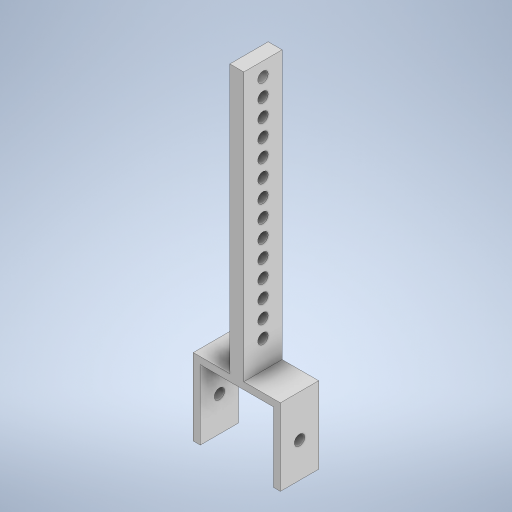
# Autodesk Inventor part: catcher
Saved by Autodesk Inventor 2024 (Build 280153000, 153)
## iProperties
Created: 2024-07-10
Part Number: catcher
Material: 일반
Document SubType Name: Modeling
Designer: Gihyeok Na
Density: 1 g/cm^3
Appearance: 기본값
Author: Gihyeok Na
Autodesk Inventor part; units mm, degrees
ref_plane "YZ Plane" through (0, 0, 0) normal (1, 0, 0) x (0, 1, 0)
ref_plane "XZ Plane" through (0, 0, 0) normal (0, 1, 0) x (-1, 0, 0)
ref_plane "XY Plane" through (0, 0, 0) normal (0, 0, 1) x (1, 0, 0)
sketch "스케치4" plane through (0, 0, 0) normal (0, 1, 0) x (-1, 0, 0)
  line L0 (-2, 5.5) -> (-2, -5.5)
  line L1 (-2, -5.5) -> (2, -5.5)
  line L2 (2, -5.5) -> (2, 5.5)
  line L3 (2, 5.5) -> (-2, 5.5)
  line L4 (-2, 5.5) -> (2, -5.5) construction
  line L5 (-2, -5.5) -> (2, 5.5) construction
  point P0 (0, 0)
  point P1 (0, 0)
  dimension "d12" = 11
  dimension "d13" = 4
  constraints: 12 end point, 3 midpoint, 2 parallel, 1 perpendicular, 1 vertical
  measures "d12" distance of L0.start L0.end
  measures "d13" distance of L1.end L0.end
extrude "돌출3" add sketch "스케치4" along normal blind 77
sketch "스케치5" plane through (0, 0, 0) normal (0, -1, 0) x (1, 0, 0)
  line L0 (-10.5, -5.5) -> (10.5, -5.5)
  line L1 (10.5, -5.5) -> (10.5, 5.5)
  line L2 (10.5, 5.5) -> (-10.5, 5.5)
  line L3 (-10.5, 5.5) -> (-10.5, -5.5)
  line L4 (-10.5, -5.5) -> (10.5, 5.5) construction
  line L5 (10.5, -5.5) -> (-10.5, 5.5) construction
  line L6 (0, 5.5) -> (0, -5.5) construction
  line L7 (10.5, 5.5) -> (12.5, 5.5)
  line L8 (12.5, 5.5) -> (12.5, -5.5)
  line L9 (12.5, -5.5) -> (10.5, -5.5)
  line L10 (-10.5, 5.5) -> (-12.5, 5.5)
  line L11 (-12.5, 5.5) -> (-12.5, -5.5)
  line L12 (-12.5, -5.5) -> (-10.5, -5.5)
  line L13 (-22.4262, 19.8) -> (40.7349, 19.8) construction
  point P0 (0, 0)
  point P1 (0, 0)
  dimension "d16" = 21
  dimension "d17" = 11
  dimension "d18" = 2
  dimension "d43" = 19.8
  constraints: 28 end point, 5 midpoint, 3 horizontal, 3 perpendicular, 2 parallel, 2 symmetric about line
  measures "d16" distance of L0.start L0.end
  measures "d17" distance of L1.end L0.end
  measures "d18" distance of L1.end L7.end
  measures "d43" distance from line of point (0, 0) L13
extrude "돌출4" add sketch "스케치5" along normal blind 2
extrude "돌출5" add sketch "스케치5" along normal blind 22 contours L12 L11 L10 L3 | L1 L7 L8 L9
sketch "스케치6" plane through (-12.5, 0, -5.5) normal (-1, 0, 0) x (0, 0, 1)
  line L0 (11, 0) -> (0, 0) projected
  line L1 (0, 0) -> (0, -22) projected
  line L2 (11, -22) -> (0, -22) projected
  line L3 (11, 0) -> (11, -22) projected
  circle A0 centre (5.5, -12) radius 1.5
  point P0 (5.5, 0)
  dimension "d23" = 3
  dimension "d24" = 10
  constraints: 1 centre point
  measures "d23" diameter of A0
  measures "d24" distance from line of A0.centre L2
extrude "돌출6" cut sketch "스케치6" against normal through all contours A0
sketch "스케치7" plane through (-2, 77, -5.5) normal (-1, 0, 0) x (0, 0, 1)
  line L0 (0, -77) -> (11, -77) projected
  line L1 (11, -77) -> (11, 0) projected
  line L2 (0, 0) -> (11, 0) projected
  line L3 (0, -77) -> (0, 0) projected
  line L4 (0, -73) -> (11, -73) construction
  line L5 (0, -4) -> (11, -4) construction
  line L6 (0, -69) -> (11, -69) construction
  circle A0 centre (5.5, -4) radius 1.5
  circle A1 centre (5.5, -69) radius 1.5
  line L7 (5.5, -69) -> (5.5, -4) construction
  circle A2 centre (5.5, -64) radius 1.5
  circle A3 centre (5.5, -59) radius 1.5
  circle A4 centre (5.5, -54) radius 1.5
  circle A5 centre (5.5, -49) radius 1.5
  circle A6 centre (5.5, -44) radius 1.5
  circle A7 centre (5.5, -39) radius 1.5
  circle A8 centre (5.5, -34) radius 1.5
  circle A9 centre (5.5, -29) radius 1.5
  circle A10 centre (5.5, -24) radius 1.5
  circle A11 centre (5.5, -19) radius 1.5
  circle A12 centre (5.5, -14) radius 1.5
  circle A13 centre (5.5, -9) radius 1.5
  point P0 (5.5, -77)
  dimension "d27" = 4
  dimension "d28" = 4
  dimension "d29" = 4
  dimension "d30" = 3
  dimension "d31" = 5.5
  dimension "d32" = 3
  dimension "d35" = 5
  constraints: 14 centre point, 8 end point, 5 point on line, 4 perpendicular, 2 midpoint, 1 vertical, 24 other
  measures "d27" distance between parallel lines of L4 L0
  measures "d28" distance between parallel lines of L5 L2
  measures "d29" distance between parallel lines of L6 L4
  measures "d30" diameter of A0
  measures "d31" distance from line of L3 L7.end
  measures "d32" diameter of A1
  measures "d35" distance of L7.start A2.centre
extrude "돌출7" cut sketch "스케치7" against normal through all contours A0 | A1 | A2 | A3 | A4 | A5 | A6 | A7 | A8 | A9 | A10 | A11 | A12 | A13
